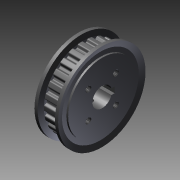
# Autodesk Inventor part: ATP25XL025-A-N10-KC90-QFC20-M3-FC45.0-TPC3_b
Saved by Autodesk Inventor 2011 SP1 (Build 150282100, 282)
## iProperties
Created: 2017-08-07
Part Number: ATP25XL025-A-N10-KC90-QFC20-M3-FC45.0-TPC3_b
Catalog Web Link: www.cadenas.de
Description: ATP__XL025, ATP__XL031, ATP__ XL037, ATP__XL050, BTP__XL025, BTP__XL031, BTP__XL037, BTP__XL050, KTP__XL025, KTP__XL031, KTP__ XL037, KTP__XL050, NTP__XL025, NTP__XL031, NTP__ XL037, NTP__XL050, MTP__XL025, MTP__ XL037, MTP__XL050, MTPB__XL025, MTPB__ XL037, MTPB__XL050, MTPP__XL025, MTPP__ XL037, MTPP__XL050, STP__XL025, STP__ XL037, STP__XL050_body-Timing Pulleys XL Type
Vendor: MISUMI
Document SubType Name: Modeling
Designer: psAdmin
Manufacturer: MISUMI
Mass: 14.4105 g
Surface Area: 66.2256 cm^2
Volume: 14.4105 cm^3
Density: 1 g/cm^3
Category: PARTsolutions
Company: MISUMI
Title: ATP25XL025-A-N10-KC90-QFC20-M3-FC45.0-TPC3
Author: Cadenas PARTsolutions
Comments: Timing Pulleys XL Type
PSOL_IDENT_0: {$CADENAS_DATA\23d-libs\misumi\metric\51_timing_pulleys\mtp_xl\mtp_xl.prj},739 {VTYP=3D},{NB=ATP25XL
PSOL_IDENT_1: 025-A-N10-KC90-QFC20-M3-FC45.0-TPC3_b},{LINA=ATP25XL025-A-N10-KC90-QFC20-M3-FC45.0-TPC3},{NN=ATP__XL
PSOL_IDENT_2: 025, ATP__XL031, ATP__ XL037, ATP__XL050, BTP__XL025, BTP__XL031, BTP__XL037, BTP__XL050, KTP__XL025
PSOL_IDENT_3: , KTP__XL031, KTP__ XL037, KTP__XL050, NTP__XL025, NTP__XL031, NTP__ XL037, NTP__XL050, MTP__XL025,
PSOL_IDENT_4: MTP__ XL037, MTP__XL050, MTPB__XL025, MTPB__ XL037, MTPB__XL050, MTPP__XL025, MTPP__ XL037, MTPP__XL
PSOL_IDENT_5: 050, STP__XL025, STP__ XL037, STP__XL050_body},{DATE=27.04.2017 02:25:46},{GEOMDATE=02.12.2016 00:36
PSOL_IDENT_6: :00},{VERSION=},{LINEID=120},{LINESUBID=-1},{WBVAR=MATP,ST,TNW,PS,SBS,DD,Z,J,Q,R,S,T,ALT1,ALT2,M,QSC
PSOL_IDENT_7: ,QFC,QTC,ALT3,K,KSC,KFC,KTC,ALT4,ZM,ZSC,ZFC,ZTC,ALT5,ALT6,ALT7,FC,ALT8,SRG,ALT9,BTC,TL,ALT10,TPC,ALT
PSOL_IDENT_8: 11,BC,ALT12,SLH}  {NB=ATP25XL025-A-N10-KC90-QFC20-M3-FC45.0-TPC3_b},{LINA=ATP25XL025-A-N10-KC90-QFC2
PSOL_IDENT_9: 0-M3-FC45.0-TPC3},{KT=DUMMY},{PN=ATP25XL025-A-N10-KC90-QFC20-M3-FC45.0-TPC3},{TYPE=ATP},{MATP=A2017}
PSOL_IDENT_10: ,{MATPALG= 'A2017','Aluminum Alloy 2000 series','S45C','1045 Carbon Steel Equivalent','SUS304','SUS3
PSOL_IDENT_11: 04' },{ST=CA},{STALG= 'CA','Clear Anodize','BA','Black Anodize','HAT','Hard Clear Anodize','ENP','El
PSOL_IDENT_12: ectroless Nickel Plating' },{NT=25},{TNW=XL025},{TNWALG= 'XL025','XL031','XL037','XL050' },{BW=6.4mm
PSOL_IDENT_13: (1/4inch)},{PS=A},{PSALG= 'A','B' },{SBS=N},{SBSALG= 'H','Round Hole','P','Round Hole + Tap','N','N
PSOL_IDENT_14: ew JIS Keywayed Bore + Tap (Standard)','NK','New JIS Keywayed Bore + Tap (width 4.0mm, height 1.8mm)'
PSOL_IDENT_15: ,'C','Old JIS Keywayed Bore + Tap','V','Stepped Hole','Y','Both Ends Stepped Hole','WB','Double Step
PSOL_IDENT_16: ped Hole' },{DD=10.00},{DDALG=[8:8/1],[10:22/1]},{DDHA=[8:12/1],12.7,[13:31/1]},{DDPA=[8:12/1],12.7,
PSOL_IDENT_17: [13:25/1]},{DDNA=[8:8/1],[10:22/1]},{DDNK=[10:10/1]},{DDCA=[10,12,15,16,18,19,20]},{DDVA=[8:12/1],12
PSOL_IDENT_18: .7,[13:29/1]},{DDY=[8:29/1]},{DDWB=[8:27/1]},{DDHB=},{DDPB=},{DDNB=},{DDCB=},{DDVFB=},{Z=0},{ZALG=[0
PSOL_IDENT_19: ]},{ZMIN=12.000},{ZAMAX=31.000},{ZBMAX=0.000},{DDZ=10.000},{J=0.0},{JALG=[0]},{JMIN=2.000},{JMAX=10}
PSOL_IDENT_20: ,{JPN=},{Q=0},{QALG=[0]},{QRMIN=12.000},{QRMAX=31},{WBQMIN=14.000},{R=0},{RALG=[0]},{WBRMAX=-2.000},
PSOL_IDENT_21: {S=0.0},{SALG=[0]},{SMAX=6.5},{T=0.0},{TALG=[0]},{TMAX=8},{SBSPN=-N10},{A=7.5},{W=12.5},{L=0},{PD=40
PSOL_IDENT_22: .43},{OD=39.92},{D=0},{DALG=30.000},{DE=35},{F=48},{E=35},{TT=1.6},{BBK=3.000},{TTK=1.4},{ALT1=KC90}
PSOL_IDENT_23: ,{ALT1ALG= '','w/o KC90 (Set Screw Angle)','KC90','with KC90 (Set Screw Angle)' },{ANG=86.400},{ALT1
PSOL_IDENT_24: PN=-KC90},{ALT2=QFC},{ALT2ALG= '','w/o Side Tapped Hole','QFC','with QFC (4 Places Side Tapped Hole)'
PSOL_IDENT_25: },{M=M3},{MALG= 'M3','M4','M5','M6','M8' },{MFTALG= 'M3','M4','M5','M6','M8' },{MSALG='M3','M4','M5'
PSOL_IDENT_26: ,'M6','M8' },{M3D=3.000},{KDML=9.500},{ML=9.500},{MUL=0.500},{PITCH=0.500},{QSC=0.0},{QSCALG=0},{QFC=
PSOL_IDENT_27: 20.0},{QFCALG=[17:28/0.5]},{QTC=0.0},{QTCALG=0},{QPCDMIN=17.000},{QPCDMINALG=17.000},{QPCDMAX=28.000
PSOL_IDENT_28: },{ALT2PN=-QFC20-M3},{TAP=6.000},{ALT3=},{ALT3ALG= '','Not applicable' },{K=0.0},{KALG=0},{KMIN=4.00
PSOL_IDENT_29: 0},{KFTMAX=8.500},{KSMAX=8.500},{KSC=0.0},{KSCALG=0},{KFC=0.0},{KFCALG=0},{KTC=0.0},{KTCALG=0},{KSCM
PSOL_IDENT_30: IN=14.000},{KPCDMIN=14.000},{KPCDMAX=31.000},{ALT3PN=},{ALT4=},{ALT4ALG= '','Not applicable' },{ALT4
PSOL_IDENT_31: MIN=20.500},{ALT4MAX=24.500},{ZM=N/A},{ZMALG= 'N/A' },{ZMFTALG= 'N/A' },{ZMSALG= 'N/A' },{ZMDD1=0.0}
PSOL_IDENT_32: ,{ZMDD2=0.0},{ZMHH=0.0},{ZSC=0.0},{ZSCALG=[0]},{ZFC=0.0},{ZFCALG=[0]},{ZTC=0.0},{ZTCALG=[0]},{ZPCDMI
PSOL_IDENT_33: N=0.000},{ZPCDMINALG=0.000},{ZPCDMAX=31.000},{ALT4PN=},{ALT5=},{ALT5ALG= '','w/o Flange not Attached'
PSOL_IDENT_34: ,'NFC','with NFC (Flange not Attached)' },{ALT5PN=},{ALT6=},{ALT6ALG= '','w/o Flange Attached on One
PSOL_IDENT_35: Side Only','RFC','with RFC (Flange Attached on The Boss Side Only)','LFC','with LFC (Flange Attache
PSOL_IDENT_36: d on The Opposite Side Only)' },{ALT6PN=},{ALT7=FC},{ALT7ALG= '','w/o FC (Flange Cut)','FC','with FC
PSOL_IDENT_37: (Flange Cut)' },{FC=45.0},{FCALG=[41:46/0.5]},{FCMIN=41.0},{FCMAX=46.0},{ALT7PN=-FC45.0},{ALT8=},{A
PSOL_IDENT_38: LT8ALG= '','Not applicable' },{ALT8ALGALG=13.000},{ALT8DD2=0.000},{ALT8MM=0.000},{ALT8NN=0.000},{QC=
PSOL_IDENT_39: 20.000},{KC=0.000},{ZC=0.000},{SRG=0.0},{SRGALG=[0]},{SRGMAX=0.000},{DD2=0.0},{MM=0.00},{NN=0.00},{A
PSOL_IDENT_40: LT8PN=},{ALT9=},{ALT9ALG= '','Not applicable' },{BTC9=11.000},{TL9=1.000},{BTC=0},{BTCALG=[0]},{TL=0
PSOL_IDENT_41: .0},{TLALG=0},{TLMIN=1.000},{TLMAX=-13.000},{BTCL=0},{BTCD=0},{ALT9PN=},{WLBCTL=12.500},{ALT10=TPC},
PSOL_IDENT_42: {ALT10ALG= '','w/o TPC (Tapped Hole Dimension)','TPC','with TPC (Tapped Hole Dimension)' },{TPC=M3},
PSOL_IDENT_43: {TPCALG= 'M3','M5' },{TPCM=4.000},{ALT10PN=-TPC3},{ALT11=},{ALT11ALG= '','Not applicable' },{BC=0.0}
PSOL_IDENT_44: ,{BCALG=0},{BCMIN=6},{BCMAX=-13},{M1WBC=6.25},{ALT11PN=},{KTT=13.56},{ALT12=},{ALT12ALG= '','w/o SLH
PSOL_IDENT_45: (Set Screw Length)','SLH','with SLH (Set Screw Length)' },{SLH=0},{SLHALG=[0]},{ALT12PN=},{AC=M3x3}
PSOL_IDENT_46: ,{M1=3.000},{M1L=3.000},{KEYA=1.000},{KEYB=0.000},{KEYM=1.000}
NN: 0.00
NT: 25
NB: ATP25XL025-A-N10-KC90-QFC20-M3-FC45.0-TPC3_b
NBSYN: $PN._b
LINA: ATP25XL025-A-N10-KC90-QFC20-M3-FC45.0-TPC3
PN: ATP25XL025-A-N10-KC90-QFC20-M3-FC45.0-TPC3
MATP: Aluminum Alloy 2000 series
ST: Clear Anodize
TNW: XL025
BW: 6.4mm (1/4inch)
PS: A
SBS: New JIS Keywayed Bore + Tap (Standard)
DD: 10.00
Z: 0
J: 0.0
Q: 0
R: 0
S: 0.0
T: 0.0
A: 7.5
W: 12.5
L: 0
PD: 40.43
OD: 39.92
D: 0
F: 48
E: 35
TT: 1.6
ALT1: with KC90 (Set Screw Angle)
ALT2: with QFC (4 Places Side Tapped Hole)
M: M3
QSC: 0.0
QFC: 20.0
QTC: 0.0
ALT3: Not applicable
K: 0.0
KSC: 0.0
KFC: 0.0
KTC: 0.0
ALT4: Not applicable
ZM: N/A
ZMDD1: 0.0
ZMDD2: 0.0
ZMHH: 0.0
ZSC: 0.0
ZFC: 0.0
ZTC: 0.0
ALT5: w/o Flange not Attached
ALT6: w/o Flange Attached on One Side Only
ALT7: with FC (Flange Cut)
FC: 45.0
ALT8: Not applicable
SRG: 0.0
DD2: 0.0
MM: 0.00
ALT9: Not applicable
BTC: 0
TL: 0.0
BTCL: 0
BTCD: 0
ALT10: with TPC (Tapped Hole Dimension)
TPC: M3
ALT11: Not applicable
BC: 0.0
ALT12: w/o SLH (Set Screw Length)
SLH: 0
AC: M3x3
SUPPLIER: MISUMI
ARTICLENO: ATP25XL025-A-N10-KC90-QFC20-M3-FC45.0-TPC3_b
BOMINFO: ATP25XL025-A-N10-KC90-QFC20-M3-FC45.0-TPC3
CREATOR: CADENAS GmbH
Autodesk Inventor part; units mm, degrees
ref_plane "YZ Plane" through (0, 0, 0) normal (1, 0, 0) x (0, 1, 0)
ref_plane "XZ Plane" through (0, 0, 0) normal (0, 1, 0) x (-1, 0, 0)
ref_plane "XY Plane" through (0, 0, 0) normal (0, 0, 1) x (1, 0, 0)
sketch "_____2" plane through (0, 0, 0) normal (0, 0, 1) x (1, 0, 0)
  line L0 (12.5, 0) -> (0, 0)
  line L1 (0, 0) -> (0, 17.5)
  line L2 (0, 17.5) -> (0.9, 17.5)
  line L3 (0.9, 17.5) -> (0.9, 19.7494)
  line L4 (0.9, 19.7494) -> (-0.128, 23.5859)
  line L5 (-0.128, 23.5859) -> (1.4175, 24)
  line L6 (1.4175, 24) -> (2.5, 19.96)
  line L7 (2.5, 19.96) -> (10, 19.96)
  line L8 (10, 19.96) -> (11.0825, 24)
  line L9 (11.0825, 24) -> (12.628, 23.5859)
  line L10 (12.628, 23.5859) -> (11.6, 19.7494)
  line L11 (11.6, 19.7494) -> (11.6, 17.5)
  line L12 (11.6, 17.5) -> (12.5, 17.5)
  line L13 (12.5, 17.5) -> (12.5, 0)
  line L14 (12.5, 0) -> (0, 0)
  constraints: 30 end point
revolve "Revolution1" add sketch "_____2" angle 360 about axis through (12.5, 0, 0) along (1, 0, 0)
sketch "Sketch2" plane through (12.5, 0, 0) normal (1, 0, 0) x (0, 0, -1)
  point P0 (0, 0)
hole "Hole1" at (12.5, 0, 0) direction (-1, 0, 0) diameter 10 depth 12.5
sketch "_____6" plane through (2.5, 0, 0) normal (1, 0, 0) x (0, 0, -1)
  arc A0 (-19.8569, 3.7879) -> (-20.1751, -1.2693) centre (0, 0) ccw
  arc A1 (-20.1751, -1.2693) -> (-19.2256, -6.2468) centre (0, 0) ccw
  arc A2 (-19.2256, -6.2468) -> (-17.0681, -10.8317) centre (0, 0) ccw
  arc A3 (-17.0681, -10.8317) -> (-13.8381, -14.7361) centre (0, 0) ccw
  arc A4 (-13.8381, -14.7361) -> (-9.7387, -17.7145) centre (0, 0) ccw
  arc A5 (-9.7387, -17.7145) -> (-5.0273, -19.5799) centre (0, 0) ccw
  arc A6 (-5.0273, -19.5799) -> (0, -20.215) centre (0, 0) ccw
  arc A7 (0, -20.215) -> (5.0273, -19.5799) centre (0, 0) ccw
  arc A8 (5.0273, -19.5799) -> (9.7387, -17.7145) centre (0, 0) ccw
  arc A9 (9.7387, -17.7145) -> (13.8381, -14.7361) centre (0, 0) ccw
  arc A10 (13.8381, -14.7361) -> (17.0681, -10.8317) centre (0, 0) ccw
  arc A11 (17.0681, -10.8317) -> (19.2256, -6.2468) centre (0, 0) ccw
  arc A12 (19.2256, -6.2468) -> (20.1751, -1.2693) centre (0, 0) ccw
  arc A13 (20.1751, -1.2693) -> (19.8569, 3.7879) centre (0, 0) ccw
  arc A14 (19.8569, 3.7879) -> (18.2911, 8.6071) centre (0, 0) ccw
  arc A15 (18.2911, 8.6071) -> (15.5759, 12.8855) centre (0, 0) ccw
  arc A16 (15.5759, 12.8855) -> (11.8821, 16.3543) centre (0, 0) ccw
  arc A17 (11.8821, 16.3543) -> (7.4416, 18.7954) centre (0, 0) ccw
  arc A18 (7.4416, 18.7954) -> (2.5336, 20.0556) centre (0, 0) ccw
  arc A19 (2.5336, 20.0556) -> (-2.5336, 20.0556) centre (0, 0) ccw
  arc A20 (-2.5336, 20.0556) -> (-7.4416, 18.7954) centre (0, 0) ccw
  arc A21 (-7.4416, 18.7954) -> (-11.8821, 16.3543) centre (0, 0) ccw
  arc A22 (-11.8821, 16.3543) -> (-15.5759, 12.8855) centre (0, 0) ccw
  arc A23 (-15.5759, 12.8855) -> (-18.2911, 8.6071) centre (0, 0) ccw
  arc A24 (-18.2911, 8.6071) -> (-19.8569, 3.7879) centre (0, 0) ccw
  arc A25 (-19.5677, 0.1331) -> (-19.955, -0.4486) centre (-19.3451, -0.4349) ccw
  arc A26 (-19.955, -0.4486) -> (-19.9206, -1.2533) centre (0, 0) ccw
  arc A27 (-19.9206, -1.2533) -> (-19.8538, -2.056) centre (0, 0) ccw
  arc A28 (-19.8538, -2.056) -> (-19.3967, -2.5845) centre (-19.2471, -1.9931) ccw
  line L0 (-19.3967, -2.5845) -> (-18.7262, -2.7542)
  arc A29 (-18.2752, -3.2391) -> (-18.7262, -2.7542) centre (-18.8758, -3.3455) ccw
  arc A30 (-18.2752, -3.2391) -> (-18.1842, -3.7159) centre (0, 0) ccw
  arc A31 (-18.425, -4.3328) -> (-18.1842, -3.7159) centre (-18.7819, -3.838) ccw
  line L1 (-18.425, -4.3328) -> (-18.986, -4.7374)
  arc A32 (-18.986, -4.7374) -> (-19.2165, -5.3971) centre (-18.6292, -5.2321) ccw
  arc A33 (-19.2165, -5.3971) -> (-18.9831, -6.168) centre (0, 0) ccw
  arc A34 (-18.9831, -6.168) -> (-18.7188, -6.9288) centre (0, 0) ccw
  arc A35 (-18.7188, -6.9288) -> (-18.1446, -7.3271) centre (-18.1467, -6.7171) ccw
  line L2 (-18.1446, -7.3271) -> (-17.4529, -7.3247)
  arc A36 (-16.8955, -7.6822) -> (-17.4529, -7.3247) centre (-17.4508, -7.9347) ccw
  arc A37 (-16.8955, -7.6822) -> (-16.6888, -8.1214) centre (0, 0) ccw
  arc A38 (-16.7687, -8.7788) -> (-16.6888, -8.1214) centre (-17.2373, -8.3883) ccw
  line L3 (-16.7687, -8.7788) -> (-17.2114, -9.3102)
  arc A39 (-17.2114, -9.3102) -> (-17.2706, -10.0065) centre (-16.7428, -9.7007) ccw
  arc A40 (-17.2706, -10.0065) -> (-16.8528, -10.6951) centre (0, 0) ccw
  arc A41 (-16.8528, -10.6951) -> (-16.4076, -11.3663) centre (0, 0) ccw
  arc A42 (-16.4076, -11.3663) -> (-15.7524, -11.6093) centre (-15.9061, -11.019) ccw
  line L4 (-15.7524, -11.6093) -> (-15.083, -11.4349)
  arc A43 (-14.4542, -11.6426) -> (-15.083, -11.4349) centre (-14.9293, -12.0252) ccw
  arc A44 (-14.4542, -11.6426) -> (-14.1448, -12.0166) centre (0, 0) ccw
  arc A45 (-14.0586, -12.6732) -> (-14.1448, -12.0166) centre (-14.6097, -12.4115) ccw
  line L5 (-14.0586, -12.6732) -> (-14.3553, -13.298)
  arc A46 (-14.3553, -13.298) -> (-14.2395, -13.9871) centre (-13.8043, -13.5596) ccw
  arc A47 (-14.2395, -13.9871) -> (-13.6636, -14.5502) centre (0, 0) ccw
  arc A48 (-13.6636, -14.5502) -> (-13.0654, -15.0896) centre (0, 0) ccw
  arc A49 (-13.0654, -15.0896) -> (-12.3704, -15.162) centre (-12.6661, -14.6285) ccw
  line L6 (-12.3704, -15.162) -> (-11.7654, -14.8267)
  arc A50 (-11.1047, -14.8714) -> (-11.7654, -14.8267) centre (-11.4697, -15.3602) ccw
  arc A51 (-11.1047, -14.8714) -> (-10.712, -15.1567) centre (0, 0) ccw
  arc A52 (-10.4653, -15.7713) -> (-10.712, -15.1567) centre (-11.0641, -15.6549) ccw
  line L7 (-10.4653, -15.7713) -> (-10.5973, -16.4502)
  arc A53 (-10.5973, -16.4502) -> (-10.3137, -17.0889) centre (-9.9985, -16.5666) ccw
  arc A54 (-10.3137, -17.0889) -> (-9.6158, -17.4911) centre (0, 0) ccw
  arc A55 (-9.6158, -17.4911) -> (-8.9023, -17.8648) centre (0, 0) ccw
  arc A56 (-8.9023, -17.8648) -> (-8.2111, -17.762) centre (-8.6302, -17.3188) ccw
  line L8 (-8.2111, -17.762) -> (-7.7086, -17.2868)
  arc A57 (-7.0575, -17.1658) -> (-7.7086, -17.2868) centre (-7.2894, -17.73) ccw
  arc A58 (-7.0575, -17.1658) -> (-6.6061, -17.3445) centre (0, 0) ccw
  arc A59 (-6.2143, -17.8784) -> (-6.6061, -17.3445) centre (-6.8233, -17.9146) ccw
  line L9 (-6.2143, -17.8784) -> (-6.1733, -18.5689)
  arc A60 (-6.1733, -18.5689) -> (-5.7398, -19.1169) centre (-5.5644, -18.5327) ccw
  arc A61 (-5.7398, -19.1169) -> (-4.9639, -19.3329) centre (0, 0) ccw
  arc A62 (-4.9639, -19.3329) -> (-4.1798, -19.5174) centre (0, 0) ccw
  arc A63 (-4.1798, -19.5174) -> (-3.5359, -19.246) centre (-4.0521, -18.921) ccw
  line L10 (-3.5359, -19.246) -> (-3.1673, -18.6607)
  arc A64 (-2.5668, -18.3817) -> (-3.1673, -18.6607) centre (-2.6511, -18.9858) ccw
  arc A65 (-2.5668, -18.3817) -> (-2.0852, -18.4425) centre (0, 0) ccw
  arc A66 (-1.5729, -18.8622) -> (-2.0852, -18.4425) centre (-2.1537, -19.0486) ccw
  line L11 (-1.5729, -18.8622) -> (-1.3615, -19.5207)
  arc A67 (-1.3615, -19.5207) -> (-0.8053, -19.9437) centre (-0.7807, -19.3342) ccw
  arc A68 (-0.8053, -19.9437) -> (0, -19.96) centre (0, 0) ccw
  arc A69 (0, -19.96) -> (0.8053, -19.9437) centre (0, 0) ccw
  arc A70 (0.8053, -19.9437) -> (1.3615, -19.5207) centre (0.7807, -19.3342) ccw
  line L12 (1.3615, -19.5207) -> (1.5729, -18.8622)
  arc A71 (2.0852, -18.4425) -> (1.5729, -18.8622) centre (2.1537, -19.0486) ccw
  arc A72 (2.0852, -18.4425) -> (2.5668, -18.3817) centre (0, 0) ccw
  arc A73 (3.1673, -18.6607) -> (2.5668, -18.3817) centre (2.6511, -18.9858) ccw
  line L13 (3.1673, -18.6607) -> (3.5359, -19.246)
  arc A74 (3.5359, -19.246) -> (4.1798, -19.5174) centre (4.0521, -18.921) ccw
  arc A75 (4.1798, -19.5174) -> (4.9639, -19.3329) centre (0, 0) ccw
  arc A76 (4.9639, -19.3329) -> (5.7398, -19.1169) centre (0, 0) ccw
  arc A77 (5.7398, -19.1169) -> (6.1733, -18.5689) centre (5.5644, -18.5327) ccw
  line L14 (6.1733, -18.5689) -> (6.2143, -17.8784)
  arc A78 (6.6061, -17.3445) -> (6.2143, -17.8784) centre (6.8233, -17.9146) ccw
  arc A79 (6.6061, -17.3445) -> (7.0575, -17.1658) centre (0, 0) ccw
  arc A80 (7.7086, -17.2868) -> (7.0575, -17.1658) centre (7.2894, -17.73) ccw
  line L15 (7.7086, -17.2868) -> (8.2111, -17.762)
  arc A81 (8.2111, -17.762) -> (8.9023, -17.8648) centre (8.6302, -17.3188) ccw
  arc A82 (8.9023, -17.8648) -> (9.6158, -17.4911) centre (0, 0) ccw
  arc A83 (9.6158, -17.4911) -> (10.3137, -17.0889) centre (0, 0) ccw
  arc A84 (10.3137, -17.0889) -> (10.5973, -16.4502) centre (9.9985, -16.5666) ccw
  line L16 (10.5973, -16.4502) -> (10.4653, -15.7713)
  arc A85 (10.712, -15.1567) -> (10.4653, -15.7713) centre (11.0641, -15.6549) ccw
  arc A86 (10.712, -15.1567) -> (11.1047, -14.8714) centre (0, 0) ccw
  arc A87 (11.7654, -14.8267) -> (11.1047, -14.8714) centre (11.4697, -15.3602) ccw
  line L17 (11.7654, -14.8267) -> (12.3704, -15.162)
  arc A88 (12.3704, -15.162) -> (13.0654, -15.0896) centre (12.6661, -14.6285) ccw
  arc A89 (13.0654, -15.0896) -> (13.6636, -14.5502) centre (0, 0) ccw
  arc A90 (13.6636, -14.5502) -> (14.2395, -13.9871) centre (0, 0) ccw
  arc A91 (14.2395, -13.9871) -> (14.3553, -13.298) centre (13.8043, -13.5596) ccw
  line L18 (14.3553, -13.298) -> (14.0586, -12.6732)
  arc A92 (14.1448, -12.0166) -> (14.0586, -12.6732) centre (14.6097, -12.4115) ccw
  arc A93 (14.1448, -12.0166) -> (14.4542, -11.6426) centre (0, 0) ccw
  arc A94 (15.083, -11.4349) -> (14.4542, -11.6426) centre (14.9293, -12.0252) ccw
  line L19 (15.083, -11.4349) -> (15.7524, -11.6093)
  arc A95 (15.7524, -11.6093) -> (16.4076, -11.3663) centre (15.9061, -11.019) ccw
  arc A96 (16.4076, -11.3663) -> (16.8528, -10.6951) centre (0, 0) ccw
  arc A97 (16.8528, -10.6951) -> (17.2706, -10.0065) centre (0, 0) ccw
  arc A98 (17.2706, -10.0065) -> (17.2114, -9.3102) centre (16.7428, -9.7007) ccw
  line L20 (17.2114, -9.3102) -> (16.7687, -8.7788)
  arc A99 (16.6888, -8.1214) -> (16.7687, -8.7788) centre (17.2373, -8.3883) ccw
  arc A100 (16.6888, -8.1214) -> (16.8955, -7.6822) centre (0, 0) ccw
  arc A101 (17.4529, -7.3247) -> (16.8955, -7.6822) centre (17.4508, -7.9347) ccw
  line L21 (17.4529, -7.3247) -> (18.1446, -7.3271)
  arc A102 (18.1446, -7.3271) -> (18.7188, -6.9288) centre (18.1467, -6.7171) ccw
  arc A103 (18.7188, -6.9288) -> (18.9831, -6.168) centre (0, 0) ccw
  arc A104 (18.9831, -6.168) -> (19.2165, -5.3971) centre (0, 0) ccw
  arc A105 (19.2165, -5.3971) -> (18.986, -4.7374) centre (18.6292, -5.2321) ccw
  line L22 (18.986, -4.7374) -> (18.425, -4.3328)
  arc A106 (18.1842, -3.7159) -> (18.425, -4.3328) centre (18.7819, -3.838) ccw
  arc A107 (18.1842, -3.7159) -> (18.2752, -3.2391) centre (0, 0) ccw
  arc A108 (18.7262, -2.7542) -> (18.2752, -3.2391) centre (18.8758, -3.3455) ccw
  line L23 (18.7262, -2.7542) -> (19.3967, -2.5845)
  arc A109 (19.3967, -2.5845) -> (19.8538, -2.056) centre (19.2471, -1.9931) ccw
  arc A110 (19.8538, -2.056) -> (19.9206, -1.2533) centre (0, 0) ccw
  arc A111 (19.9206, -1.2533) -> (19.955, -0.4486) centre (0, 0) ccw
  arc A112 (19.955, -0.4486) -> (19.5677, 0.1331) centre (19.3451, -0.4349) ccw
  line L24 (19.5677, 0.1331) -> (18.9237, 0.3855)
  arc A113 (18.537, 0.9231) -> (18.9237, 0.3855) centre (19.1463, 0.9534) ccw
  arc A114 (18.537, 0.9231) -> (18.5066, 1.4075) centre (0, 0) ccw
  arc A115 (18.8228, 1.9894) -> (18.5066, 1.4075) centre (19.1148, 1.4538) ccw
  line L25 (18.8228, 1.9894) -> (19.4301, 2.3205)
  arc A116 (19.4301, 2.3205) -> (19.7414, 2.9461) centre (19.1381, 2.856) ccw
  arc A117 (19.7414, 2.9461) -> (19.6065, 3.7401) centre (0, 0) ccw
  arc A118 (19.6065, 3.7401) -> (19.4396, 4.5281) centre (0, 0) ccw
  arc A119 (19.4396, 4.5281) -> (18.9198, 4.9952) centre (18.8455, 4.3897) ccw
  line L26 (18.9198, 4.9952) -> (18.2333, 5.0795)
  arc A120 (17.7251, 5.504) -> (18.2333, 5.0795) centre (18.3077, 5.6849) ccw
  arc A121 (17.7251, 5.504) -> (17.5751, 5.9657) centre (0, 0) ccw
  arc A122 (17.7367, 6.6079) -> (17.5751, 5.9657) centre (18.1527, 6.1618) ccw
  line L27 (17.7367, 6.6079) -> (18.2426, 7.0796)
  arc A123 (18.2426, 7.0796) -> (18.3885, 7.763) centre (17.8265, 7.5257) ccw
  arc A124 (18.3885, 7.763) -> (18.0603, 8.4986) centre (0, 0) ccw
  arc A125 (18.0603, 8.4986) -> (17.7028, 9.2203) centre (0, 0) ccw
  arc A126 (17.7028, 9.2203) -> (17.0832, 9.5434) centre (17.1618, 8.9385) ccw
  line L28 (17.0832, 9.5434) -> (16.3973, 9.4543)
  arc A127 (15.7994, 9.7392) -> (16.3973, 9.4543) centre (16.3187, 10.0593) ccw
  arc A128 (15.7994, 9.7392) -> (15.5393, 10.149) centre (0, 0) ccw
  arc A129 (15.5362, 10.8112) -> (15.5393, 10.149) centre (16.0501, 10.4826) ccw
  line L29 (15.5362, 10.8112) -> (15.9088, 11.3939)
  arc A130 (15.9088, 11.3939) -> (15.8802, 12.0921) centre (15.3949, 11.7226) ccw
  arc A131 (15.8802, 12.0921) -> (15.3794, 12.723) centre (0, 0) ccw
  arc A132 (15.3794, 12.723) -> (14.8536, 13.3331) centre (0, 0) ccw
  arc A133 (14.8536, 13.3331) -> (14.1731, 13.492) centre (14.3997, 12.9256) ccw
  line L30 (14.1731, 13.492) -> (13.5309, 13.2351)
  arc A134 (12.881, 13.3624) -> (13.5309, 13.2351) centre (13.3044, 13.8015) ccw
  arc A135 (12.881, 13.3624) -> (12.5272, 13.6946) centre (0, 0) ccw
  arc A136 (12.3594, 14.3353) -> (12.5272, 13.6946) centre (12.9389, 14.1447) ccw
  line L31 (12.3594, 14.3353) -> (12.5755, 14.9923)
  arc A137 (12.5755, 14.9923) -> (12.3741, 15.6615) centre (11.996, 15.1829) ccw
  arc A138 (12.3741, 15.6615) -> (11.7322, 16.148) centre (0, 0) ccw
  arc A139 (11.7322, 16.148) -> (11.0711, 16.6082) centre (0, 0) ccw
  arc A140 (11.0711, 16.6082) -> (10.3725, 16.5929) centre (10.7328, 16.1006) ccw
  line L32 (10.3725, 16.5929) -> (9.8144, 16.1843)
  arc A141 (9.1533, 16.1459) -> (9.8144, 16.1843) centre (9.4541, 16.6766) ccw
  arc A142 (9.1533, 16.1459) -> (8.7279, 16.3798) centre (0, 0) ccw
  arc A143 (8.4061, 16.9586) -> (8.7279, 16.3798) centre (9.0147, 16.9181) ccw
  line L33 (8.4061, 16.9586) -> (8.4519, 17.6487)
  arc A144 (8.4519, 17.6487) -> (8.0905, 18.2468) centre (7.8433, 17.6891) ccw
  arc A145 (8.0905, 18.2468) -> (7.3478, 18.5583) centre (0, 0) ccw
  arc A146 (7.3478, 18.5583) -> (6.593, 18.8397) centre (0, 0) ccw
  arc A147 (6.593, 18.8397) -> (5.9202, 18.6511) centre (6.3916, 18.2639) ccw
  line L34 (5.9202, 18.6511) -> (5.4812, 18.1166)
  arc A148 (4.8504, 17.915) -> (5.4812, 18.1166) centre (5.0098, 18.5038) ccw
  arc A149 (4.8504, 17.915) -> (4.3802, 18.0357) centre (0, 0) ccw
  arc A150 (3.9246, 18.5163) -> (4.3802, 18.0357) centre (4.5242, 18.6285) ccw
  line L35 (3.9246, 18.5163) -> (3.7973, 19.1962)
  arc A151 (3.7973, 19.1962) -> (3.2986, 19.6856) centre (3.1977, 19.0839) ccw
  arc A152 (3.2986, 19.6856) -> (2.5017, 19.8026) centre (0, 0) ccw
  arc A153 (2.5017, 19.8026) -> (1.7007, 19.8874) centre (0, 0) ccw
  arc A154 (1.7007, 19.8874) -> (1.0959, 19.5374) centre (1.6487, 19.2796) ccw
  line L36 (1.0959, 19.5374) -> (0.8035, 18.9106)
  arc A155 (0.2427, 18.5584) -> (0.8035, 18.9106) centre (0.2507, 19.1684) ccw
  arc A156 (0.2427, 18.5584) -> (-0.2427, 18.5584) centre (0, 0) ccw
  arc A157 (-0.8035, 18.9106) -> (-0.2427, 18.5584) centre (-0.2507, 19.1684) ccw
  line L37 (-0.8035, 18.9106) -> (-1.0959, 19.5374)
  arc A158 (-1.0959, 19.5374) -> (-1.7007, 19.8874) centre (-1.6487, 19.2796) ccw
  arc A159 (-1.7007, 19.8874) -> (-2.5017, 19.8026) centre (0, 0) ccw
  arc A160 (-2.5017, 19.8026) -> (-3.2986, 19.6856) centre (0, 0) ccw
  arc A161 (-3.2986, 19.6856) -> (-3.7973, 19.1962) centre (-3.1977, 19.0839) ccw
  line L38 (-3.7973, 19.1962) -> (-3.9246, 18.5163)
  arc A162 (-4.3802, 18.0357) -> (-3.9246, 18.5163) centre (-4.5242, 18.6285) ccw
  arc A163 (-4.3802, 18.0357) -> (-4.8504, 17.915) centre (0, 0) ccw
  arc A164 (-5.4812, 18.1166) -> (-4.8504, 17.915) centre (-5.0098, 18.5038) ccw
  line L39 (-5.4812, 18.1166) -> (-5.9202, 18.6511)
  arc A165 (-5.9202, 18.6511) -> (-6.593, 18.8397) centre (-6.3916, 18.2639) ccw
  arc A166 (-6.593, 18.8397) -> (-7.3478, 18.5583) centre (0, 0) ccw
  arc A167 (-7.3478, 18.5583) -> (-8.0905, 18.2468) centre (0, 0) ccw
  arc A168 (-8.0905, 18.2468) -> (-8.4519, 17.6487) centre (-7.8433, 17.6891) ccw
  line L40 (-8.4519, 17.6487) -> (-8.4061, 16.9586)
  arc A169 (-8.7279, 16.3798) -> (-8.4061, 16.9586) centre (-9.0147, 16.9181) ccw
  arc A170 (-8.7279, 16.3798) -> (-9.1533, 16.1459) centre (0, 0) ccw
  arc A171 (-9.8144, 16.1843) -> (-9.1533, 16.1459) centre (-9.4541, 16.6766) ccw
  line L41 (-9.8144, 16.1843) -> (-10.3725, 16.5929)
  arc A172 (-10.3725, 16.5929) -> (-11.0711, 16.6082) centre (-10.7328, 16.1006) ccw
  arc A173 (-11.0711, 16.6082) -> (-11.7322, 16.148) centre (0, 0) ccw
  arc A174 (-11.7322, 16.148) -> (-12.3741, 15.6615) centre (0, 0) ccw
  arc A175 (-12.3741, 15.6615) -> (-12.5755, 14.9923) centre (-11.996, 15.1829) ccw
  line L42 (-12.5755, 14.9923) -> (-12.3594, 14.3353)
  arc A176 (-12.5272, 13.6946) -> (-12.3594, 14.3353) centre (-12.9389, 14.1447) ccw
  arc A177 (-12.5272, 13.6946) -> (-12.881, 13.3624) centre (0, 0) ccw
  arc A178 (-13.5309, 13.2351) -> (-12.881, 13.3624) centre (-13.3044, 13.8015) ccw
  line L43 (-13.5309, 13.2351) -> (-14.1731, 13.492)
  arc A179 (-14.1731, 13.492) -> (-14.8536, 13.3331) centre (-14.3997, 12.9256) ccw
  arc A180 (-14.8536, 13.3331) -> (-15.3794, 12.723) centre (0, 0) ccw
  arc A181 (-15.3794, 12.723) -> (-15.8802, 12.0921) centre (0, 0) ccw
  arc A182 (-15.8802, 12.0921) -> (-15.9088, 11.3939) centre (-15.3949, 11.7226) ccw
  line L44 (-15.9088, 11.3939) -> (-15.5362, 10.8112)
  arc A183 (-15.5393, 10.149) -> (-15.5362, 10.8112) centre (-16.0501, 10.4826) ccw
  arc A184 (-15.5393, 10.149) -> (-15.7994, 9.7392) centre (0, 0) ccw
  arc A185 (-16.3973, 9.4543) -> (-15.7994, 9.7392) centre (-16.3187, 10.0593) ccw
  line L45 (-16.3973, 9.4543) -> (-17.0832, 9.5434)
  arc A186 (-17.0832, 9.5434) -> (-17.7028, 9.2203) centre (-17.1618, 8.9385) ccw
  arc A187 (-17.7028, 9.2203) -> (-18.0603, 8.4986) centre (0, 0) ccw
  arc A188 (-18.0603, 8.4986) -> (-18.3885, 7.763) centre (0, 0) ccw
  arc A189 (-18.3885, 7.763) -> (-18.2426, 7.0796) centre (-17.8265, 7.5257) ccw
  line L46 (-18.2426, 7.0796) -> (-17.7367, 6.6079)
  arc A190 (-17.5751, 5.9657) -> (-17.7367, 6.6079) centre (-18.1527, 6.1618) ccw
  arc A191 (-17.5751, 5.9657) -> (-17.7251, 5.504) centre (0, 0) ccw
  arc A192 (-18.2333, 5.0795) -> (-17.7251, 5.504) centre (-18.3077, 5.6849) ccw
  line L47 (-18.2333, 5.0795) -> (-18.9198, 4.9952)
  arc A193 (-18.9198, 4.9952) -> (-19.4396, 4.5281) centre (-18.8455, 4.3897) ccw
  arc A194 (-19.4396, 4.5281) -> (-19.6065, 3.7401) centre (0, 0) ccw
  arc A195 (-19.6065, 3.7401) -> (-19.7414, 2.9461) centre (0, 0) ccw
  arc A196 (-19.7414, 2.9461) -> (-19.4301, 2.3205) centre (-19.1381, 2.856) ccw
  line L48 (-19.4301, 2.3205) -> (-18.8228, 1.9894)
  arc A197 (-18.5066, 1.4075) -> (-18.8228, 1.9894) centre (-19.1148, 1.4538) ccw
  arc A198 (-18.5066, 1.4075) -> (-18.537, 0.9231) centre (0, 0) ccw
  arc A199 (-18.9237, 0.3855) -> (-18.537, 0.9231) centre (-19.1463, 0.9534) ccw
  line L49 (-18.9237, 0.3855) -> (-19.5677, 0.1331)
  constraints: 400 point on circle, 200 centre point, 100 end point
extrude "Extrusion1" cut sketch "_____6" along normal blind 7.5
sketch "_____43" plane through (0, 0, 0) normal (1, 0, 0) x (0, 0, -1)
  line L0 (-1.5, 6.4) -> (-1.5, 0)
  line L1 (-1.5, 0) -> (1.5, 0)
  line L2 (1.5, 0) -> (1.5, 6.4)
  line L3 (1.5, 6.4) -> (-1.5, 6.4)
  constraints: 8 end point
extrude "Extrusion2" cut sketch "_____43" along normal blind 12.5
sketch "_____14" plane through (0, 0, 0) normal (0, 0, 1) x (1, 0, 0)
  line L0 (500, 0) -> (-500, 0)
  line L1 (-12.5, 48) -> (-12.5, 22.5)
  line L2 (-12.5, 22.5) -> (25, 22.5)
  line L3 (25, 22.5) -> (25, 48)
  line L4 (25, 48) -> (-12.5, 48)
  constraints: 10 end point
revolve "Revolution2" cut sketch "_____14" angle 360 about axis through (500, 0, 0) along (1, 0, 0)
sketch "_____15" plane through (6.25, 0, 0) normal (1, 0, 0) x (0, 0, -1)
  line L0 (0, 0) -> (0, 19.96)
  line L1 (0, 19.96) -> (1.2295, 19.96)
  line L2 (1.2295, 19.96) -> (1.2295, 0)
  line L3 (1.2295, 0) -> (0, 0)
  line L4 (0, 0) -> (0, 19.96)
  constraints: 10 end point
revolve "Revolution3" cut sketch "_____15" angle 360 about axis through (6.25, 0, 0) along (0, -1, 0)
thread "Thread1" size "M3x0.5" class "6H" standard "ISO Metric profile" length 13.56
sketch "_____16" plane through (6.25, 0, 0) normal (1, 0, 0) x (0, 0, -1)
  line L0 (0, 0) -> (19.9206, 1.2533)
  line L1 (19.9206, 1.2533) -> (19.9978, 0.0262)
  line L2 (19.9978, 0.0262) -> (0.0772, -1.2271)
  line L3 (0.0772, -1.2271) -> (0, 0)
  line L4 (0, 0) -> (19.9206, 1.2533)
  constraints: 10 end point
revolve "Revolution4" cut sketch "_____16" angle 360 about axis through (6.25, 0, 0) along (0, -0.0627905, 0.9980267)
thread "Thread2" size "M3x0.5" class "6H" standard "ISO Metric profile" length 14.96
sketch "Sketch8" plane through (12.5, 0, 0) normal (1, 0, 0) x (0, 0, -1)
  point P0 (7.0711, 7.0711)
hole "Hole2" at (12.5, 7.0711, -7.0711) direction (-1, 0, 0) diameter 2.459 depth 8.7901 tip angle 120 countersink diameter 3 countersink angle 90 thread size "M3x0.5" class "6H" standard "ISO Metric profile"
pattern_linear "Rectangular Pattern1" count 2 spacing 14.1421 along (0, 0, 1) count 2 spacing 14.1421 along (0, -1, 0) of "Hole2"
ref_plane "to_screw1_XY" through (6.25, 6.4, 0) normal (0, 1, 0) x (1, 0, 0)
ref_plane "to_screw1_YZ" through (6.25, 6.4, 0) normal (1, 0, 0) x (0, 0, -1)
ref_plane "to_screw1_ZX" through (6.25, 6.4, 0) normal (0, 0, -1) x (0, 1, 0)
ref_plane "to_screw2_XY" through (6.25, 0.314, -4.9901) normal (0, 0.0627905, -0.9980267) x (1, 0, 0)
ref_plane "to_screw2_YZ" through (6.25, 0.314, -4.9901) normal (1, 0, 0) x (0, -0.9980267, -0.0627905)
ref_plane "to_screw2_ZX" through (6.25, 0.314, -4.9901) normal (0, -0.9980267, -0.0627905) x (0, 0.0627905, -0.9980267)
body "Solid1"
